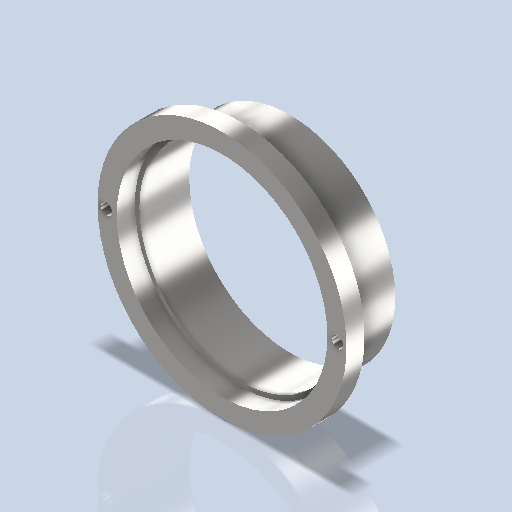
# Autodesk Inventor part: 4
Saved by Autodesk Inventor 2024.2 (Build 282272000, 272)
## iProperties
Created: 2024-05-04
Part Number: 4
Material: Stahl, Kohlenstoff
Document SubType Name: Modeling
Designer: Fabri
Density: 7.85 g/cm^3
Appearance: Halbpoliert
Author: Fabri
Autodesk Inventor part; units mm, degrees
ref_plane "YZ Plane" through (0, 0, 0) normal (1, 0, 0) x (0, 1, 0)
ref_plane "XZ Plane" through (0, 0, 0) normal (0, 1, 0) x (-1, 0, 0)
ref_plane "XY Plane" through (0, 0, 0) normal (0, 0, 1) x (1, 0, 0)
sketch "Skizze1" plane through (0, 0, 0) normal (0, 1, 0) x (-1, 0, 0)
  circle A0 centre (0, 0) radius 137.5
  circle A1 centre (0, 0) radius 116.25
  circle A2 centre (0, 0) radius 111.25
  dimension "d0" = 275
  dimension "d1" = 232.5
  dimension "d2" = 222.5
  constraints: 3 centre point, 3 coincident
  measures "d0" diameter of A0
  measures "d1" diameter of A1
  measures "d2" diameter of A2
extrude "Extrusion1" add sketch "Skizze1" against normal blind 20 contours A0
extrude "Extrusion2" add sketch "Skizze1" along normal blind 55 contours A1
sketch "Skizze2" plane through (0, 0, 0) normal (0, 1, 0) x (1, 0, 0)
  point P0 (0, 0)
  point P1 (-127.5, 0)
  point P2 (127.5, 0)
  dimension "d14" = 127.5
  dimension "d15" = 127.5
  constraints: 2 horizontal alignment
  measures "d14" distance of point (0, 0) point (-127.5, 0)
  measures "d15" distance of point (0, 0) point (127.5, 0)
hole "Bohrung1" at (-127.5, 0, 0) at (127.5, 0, 0) direction (0, -1, 0) diameter 12.5 depth 20
